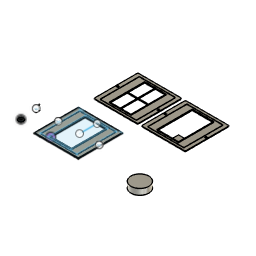
Window test bench 3D scanner (Autodesk Fusion 360 design; units mm, degrees)
Autodesk Fusion 360 part; units mm, degrees
note: some values were not read from the file. Set by a fixed rule: which sketch regions a step uses.
sketch "Sketch1" plane through (0, 0, 0) normal (0, 0, 1) x (1, 0, 0)
  line L0 (0, 0) -> (35, 0)
  line L1 (35, 0) -> (35, 58)
  line L2 (35, 58) -> (0, 58)
  line L3 (0, 58) -> (0, 0)
  line L4 (19, 59) -> (19, 29.5)
  circle A0 centre (-16.8269, 29.5) radius 0.5
  circle A1 centre (51.9731, 29.4986) radius 0.5
  circle A2 centre (-16.8269, 29.5) radius 1.75
  circle A3 centre (51.9731, 29.4986) radius 1.75
  line L5 (-10, 66) -> (48, 66)
  line L6 (48, -8) -> (-10, -8)
  line L7 (48, -8) -> (54.4, -8)
  line L8 (54.4, -8) -> (54.4, 66)
  line L9 (-10, -8) -> (-19.4, -8)
  line L10 (-19.4, -8) -> (-19.4, 65.9685)
  line L11 (-10, 66) -> (-19.4, 65.9685)
  line L12 (48, 66) -> (54.4, 66)
  dimension "d1" = 35
  dimension "d2" = 58
  dimension "d9" = 1
  dimension "d10" = 1
  dimension "d11" = 68.8
  dimension "d12" = 3.5
  dimension "d13" = 3.5
  dimension "d16" = 8
  dimension "d25" = 19.4
  dimension "d26" = 19.4
  dimension "d27" = 8
  dimension "d31" = 36.5
  dimension "d32" = 36.5014
  constraint horizontal L0
  constraint vertical L1
  constraint horizontal L2
  constraint vertical L3
  constraint coincident L0.start L3.end
  constraint perpendicular L2 L4
  constraint concentric A0 A2
  constraint concentric A1 A3
  constraint horizontal L7
  constraint vertical L8
  constraint horizontal L9
  constraint vertical L10
  measures "d1" distance of L0.start L0.end
  measures "d2" distance of L0.start L2.end
  measures "d9" diameter of A0
  measures "d10" diameter of A1
  measures "d11" distance of A0.centre A1.centre
  measures "d12" diameter of A2
  measures "d13" diameter of A3
  measures "d16" distance of L2 L5
  measures "d25" distance of L3 L10
  measures "d26" distance of L1 L8
  measures "d27" distance of L0 L6
  measures "d31" distance of A0.centre L5
  measures "d32" distance of A1.centre L5
extrude "Extrude2" add sketch "Sketch1" along normal blind 1 contours L5 L6 L7 L8 L9 L10 L11 L12 makes body 1
sketch "Sketch2" plane through (0, 0, 0) normal (0, 0, 1) x (1, 0, 0)
  circle A0 centre (-50, 0) radius 4
  dimension "d19" = 8
  measures "d19" diameter of A0
extrude "Extrude3" add sketch "Sketch2" along normal blind 1 separate body makes body 2
sketch "Sketch3" plane through (0, 0, 1) normal (0, 0, 1) x (-1, 0, 0)
  circle A0 centre (50, 0) radius 4
  circle A1 centre (50, 0) radius 0.5
  dimension "d22" = 1
  constraint concentric A0 A1
  measures "d22" diameter of A1
extrude "Extrude4" add sketch "Sketch3" along normal blind 3 contours A1 bodies 2
fillet "Fillet1" radius 1.5 4 edges at (54.4, -8, 0.5) (-19.4, 65.9685, 0.5) (54.4, 66, 0.5) (-19.4, -8, 0.5) on bodies 1
sketch "Sketch4" plane through (0, 0, 1) normal (0, 0, 1) x (-1, 0, 0)
  arc A0 (19.4, 6.5) -> (17.9, 8) centre (17.9, 6.5) ccw
  line L0 (17.9, 8) -> (-52.9, 8)
  arc A1 (-52.9, 8) -> (-54.4, 6.5) centre (-52.9, 6.5) ccw
  line L1 (-54.4, 6.5) -> (-54.4, -64.5)
  arc A2 (-54.4, -64.5) -> (-52.9, -66) centre (-52.9, -64.5) ccw
  line L2 (-52.9, -66) -> (-48, -66)
  line L3 (-48, -66) -> (10, -66)
  line L4 (10, -66) -> (17.905, -65.9735)
  arc A3 (17.905, -65.9735) -> (19.4, -64.4735) centre (17.9, -64.4735) ccw
  line L5 (19.4, -64.4735) -> (19.4, 6.5)
  line L6 (0, 0) -> (0, -58)
  line L7 (0, -58) -> (-35, -58)
  line L8 (-35, -58) -> (-35, 0)
  line L9 (-35, 0) -> (0, 0)
  circle A4 centre (-51.9731, -29.4986) radius 1.75
  circle A5 centre (16.8269, -29.5) radius 1.75
  line L10 (13, 4) -> (-48, 4)
  line L11 (-48, 4) -> (-48, -62)
  line L12 (-48, -62) -> (13, -62)
  line L13 (13, -62) -> (13, 4)
  line L14 (1, -59) -> (-36, -59)
  line L15 (-36, -59) -> (-36, 1)
  line L16 (-36, 1) -> (1, 1)
  line L17 (1, 1) -> (1, -59)
  constraint horizontal L10
  constraint vertical L11
  constraint horizontal L12
  constraint vertical L13
  constraint horizontal L14
  constraint vertical L15
  constraint horizontal L16
  constraint vertical L17
extrude "Extrude5" cut sketch "Sketch4" against normal blind 0.5 contours L10 L11 L12 L13 bodies 1
sketch "Sketch5" plane through (0, 0, 0) normal (0, 0, 1) x (1, 0, 0)
  circle A0 centre (-54, 29.5) radius 1
  circle A1 centre (-54, 29.5) radius 2
  dimension "d37" = 2
  dimension "d40" = 4
  constraint concentric A0 A1
  measures "d37" diameter of A0
  measures "d40" diameter of A1
extrude "Extrude6" add sketch "Sketch5" along normal blind 8 separate body contours A0 makes body 3
extrude "Extrude7" add sketch "Sketch5" against normal blind 5 separate body contours A0 makes body 4
move_face "MoveFace1" to x (1, 0, 0) y (0, 1, 0) z (0, 0, 1) at (5, 0, 0) 1 faces at (-53.0012, 29.4502, 5.3333) on bodies 3
extrude "Extrude8" add sketch "Sketch5" along normal blind 0.2 separate body makes body 5
extrude "Extrude9" cut 1 faces at (-52.3408, 29.4006, 0.2) along direction (0, 0, -1) blind 0.1 on bodies 5 bodies 5
sketch "Sketch6" plane through (0, 0, 1) normal (0, 0, 1) x (-1, 0, 0)
  circle A0 centre (-150, 0) radius 15
  dimension "d47" = 30
  measures "d47" diameter of A0
extrude "Extrude10" add sketch "Sketch6" along normal blind 10 separate body makes body 6
copy_body "CopyPasteBodies1" bodies 1 makes body 7
move_body "Move1" bodies 7 to x (1, 0, 0) y (0, 1, 0) z (0, 0, 1) at (0, 100, 0)
copy_body "CopyPasteBodies2" bodies 1 makes body 8
move_body "Move2" bodies 8 to x (1, 0, 0) y (0, 1, 0) z (0, 0, 1) at (80, 100, 0)
sketch "Sketch7" plane through (0, 0, 0.5) normal (0, 0, 1) x (-1, 0, 0)
  line L0 (-36, -99) -> (1, -99)
  line L1 (1, -99) -> (1, -159)
  line L2 (1, -159) -> (-36, -159)
  line L3 (-36, -159) -> (-36, -99)
  line L4 (13, -162) -> (13, -96)
  line L5 (13, -96) -> (-48, -96)
  line L6 (-48, -96) -> (-48, -162)
  line L7 (-48, -162) -> (13, -162)
  line L8 (1, -159) -> (1, -129)
  line L9 (-35, -129.5) -> (-35, -128.5)
  line L10 (0, -128.5) -> (0, -129.5)
  line L11 (-18, -158) -> (-17, -158)
  line L12 (-17, -100) -> (-18, -100)
  line L13 (-35, -128.5) -> (-18, -128.5)
  line L14 (-17, -128.5) -> (0, -128.5)
  line L15 (-17, -158) -> (-17, -129.5)
  line L16 (-17, -128.5) -> (-17, -100)
  line L17 (1, -129.5) -> (-17, -129.5)
  line L18 (-18, -129.5) -> (-35, -129.5)
  line L19 (-18, -100) -> (-18, -128.5)
  line L20 (-18, -129.5) -> (-18, -158)
  dimension "d50" = 1
  constraint coincident L1.end L2.start
  constraint midpoint L1 L8.end
  constraint coincident L8 L17.start
  constraint perpendicular L3 L17
  constraint perpendicular L3 L13
  constraint coincident L10.end L17
  constraint perpendicular L10 L17
  constraint horizontal L11
  constraint vertical L15
  constraint horizontal L12
  constraint vertical L19
  constraint coincident L14.start L15
  constraint collinear L13 L14
  constraint collinear L15 L16
  constraint coincident L18.start L19
  constraint collinear L17 L18
  constraint collinear L19 L20
  measures "d50" distance of L11.start L11.end
extrude "Extrude11" add sketch "Sketch7" along normal blind 0.5 and the other way blind 0.5 contours L9 L10 L11 L12 L13 L14 L15 L16 L17 L18 L19 L20 bodies 7
sketch "Sketch8" plane through (0, 0, 1) normal (0, 0, 1) x (-1, 0, 0)
  line L0 (-79, -159) -> (-79, -99)
  line L1 (-79, -99) -> (-116, -99)
  line L2 (-116, -99) -> (-116, -159)
  line L3 (-116, -159) -> (-79, -159)
  line L4 (-80, -100) -> (-80, -158)
  line L5 (-80, -158) -> (-115, -158)
  line L6 (-115, -158) -> (-115, -100)
  line L7 (-115, -100) -> (-80, -100)
  line L8 (-115, -100) -> (-105, -100)
  line L9 (-105, -100) -> (-105, -110)
  line L10 (-105, -110) -> (-115, -110)
  line L11 (-115, -110) -> (-115, -100)
  dimension "d55" = 10
  dimension "d56" = 10
  constraint horizontal L8
  constraint vertical L9
  constraint horizontal L10
  constraint vertical L11
  constraint coincident L6.end L7.start
  measures "d55" distance of L6.end L8.end
  measures "d56" distance of L6.end L10.end
extrude "Extrude12" add sketch "Sketch8" against normal blind 1 separate body contours L6 L7 L8 L9 L10 L11 makes body 9
